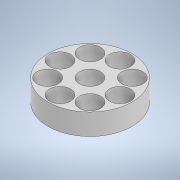
# Autodesk Inventor part: vial holder
Saved by Autodesk Inventor 2022 (Build 260153000, 153)
## iProperties
Created: 2022-08-04
Part Number: vial holder
Material: Generic
Document SubType Name: Modeling
Designer: efred
Density: 1 g/cm^3
Appearance: Default
Author: efred
Autodesk Inventor part; units mm, degrees
ref_plane "YZ Plane" through (0, 0, 0) normal (1, 0, 0) x (0, 1, 0)
ref_plane "XZ Plane" through (0, 0, 0) normal (0, 1, 0) x (-1, 0, 0)
ref_plane "XY Plane" through (0, 0, 0) normal (0, 0, 1) x (1, 0, 0)
sketch "Sketch1" plane through (0, 0, 0) normal (0, 1, 0) x (-1, 0, 0)
  circle A0 centre (0, 0) radius 27.5 construction
  circle A1 centre (42.5, 0) radius 15
  circle A2 centre (30.052, 30.052) radius 15
  circle A3 centre (0, 42.5) radius 15
  circle A4 centre (-30.052, 30.052) radius 15
  circle A5 centre (-42.5, 0) radius 15
  circle A6 centre (0, 0) radius 59.5
  circle A7 centre (0, 0) radius 15
  circle A8 centre (-30.052, -30.052) radius 15
  circle A9 centre (0, -42.5) radius 15
  circle A10 centre (30.052, -30.052) radius 15
  point P0 (19.4454, 19.4454)
  point P1 (27.5, 0)
  point P2 (-27.5, 0)
  point P3 (-19.4454, 19.4454)
  point P4 (0, 27.5)
  dimension "d0" = 55
  dimension "d1" = 30
  dimension "d4" = 360
  dimension "d6" = 32
  dimension "d19" = 30
  constraints: 11 centre point, 2 coincident, 1 horizontal alignment, 1 tangent, 17 other
  measures "d0" diameter of A0
  measures "d1" diameter of A1
  measures "d6" radial gap between concentric circles of A0 A6
  measures "d19" diameter of A7
extrude "Extrusion1" add sketch "Sketch1" along normal blind 30
body "Solid1"
